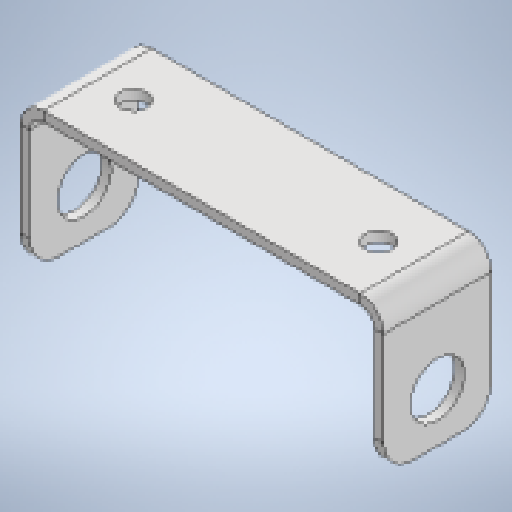
# Autodesk Inventor part: TKS 3525 FDS diam support
Saved by Autodesk Inventor 2025 (Build 290162010, 162A)
## iProperties
Created: 2025-06-24
Part Number: TKS 3525 FDS diam support
Material: Stainless Steel
Document SubType Name: Sheet Metal
Designer: admin
Mass: 14.3451 g
Surface Area: 20.2627 cm^2
Volume: 1.79313 cm^3
Density: 8 g/cm^3
Flat Pattern Width: 12.6404 cm
Flat Pattern Length: 2.2 cm
Flat Pattern Area: 27.8089 cm^2
Sheet Metal Rule: AISI304 2mm Die16
Sheet Metal Width: 126,404 mm
Sheet Metal Length: 22,000 mm
Sheet Metal Area: 2780,888 mm^2
Appearance: Default
Author: user
Autodesk Inventor part; units mm, degrees
ref_plane "YZ Plane" through (0, 0, 0) normal (1, 0, 0) x (0, 1, 0)
ref_plane "XZ Plane" through (0, 0, 0) normal (0, 1, 0) x (-1, 0, 0)
ref_plane "XY Plane" through (0, 0, 0) normal (0, 0, 1) x (1, 0, 0)
sketch "Sketch1" plane through (0, 0, 0) normal (0, 0, 1) x (1, 0, 0)
  line L0 (-35, -11) -> (35, -11)
  line L1 (35, -11) -> (35, 11)
  line L2 (35, 11) -> (-35, 11)
  line L3 (-35, 11) -> (-35, -11)
  line L4 (-35, -11) -> (35, 11) construction
  line L5 (35, -11) -> (-35, 11) construction
  circle A0 centre (-25, 0) radius 2.75
  circle A1 centre (25, 0) radius 2.75
  line L6 (0, 11) -> (0, -18.7198) construction
  point P0 (0, 0)
  dimension "d154" = 70
  dimension "d155" = 22
  dimension "d197" = 50
  dimension "d198" = 5.5
  measures "d154" distance of L1.end L2.end
  measures "d155" distance of L0.end L1.end
  measures "d197" distance of A1.centre A0.centre
  measures "d198" diameter of A0
extrude "Plate5" add sketch "Sketch1" along normal blind 2
sketch "Sketch10" plane through (-37, 11, 2) normal (1, 0, 0) x (0, 1, 0)
  line L0 (-22, 0) -> (0, 0)
  line L1 (0, 0) -> (0, -30)
  line L2 (0, -30) -> (-22, -30)
  line L3 (-22, -30) -> (-22, 0)
  constraints: 8 end point
edge flange "Flange4" height 30 angle 90 thickness 2 bend radius 2.75 thickness toward (1, 0, 0) relief round relief width 2 relief depth 1 corner gap 2.75 corner form 0 edges at (-35, 0, 0) (35, 0, 0) wall of the first edge with corners at (-37, -11, 2) (-37, 11, 2) (-37, 11, -28) (-37, -11, -28)
bend "Bend4"
corner "Corner4"
sketch "Sketch11" plane through (-35, -11, -28) normal (1, 0, 0) x (0, 0, -1)
  line L0 (-25.25, 22) -> (-25.25, 0) construction
  line L1 (-25.25, 0) -> (0, 0) construction
  line L2 (0, 0) -> (0, 22) construction
  line L3 (-25.25, 22) -> (0, 22) construction
  circle A0 centre (-10, 11) radius 5.5
  point P0 (-28, 11)
  point P1 (0, 11)
  dimension "d192" = 11
  dimension "d193" = 10
  constraints: 1 centre point, 1 horizontal alignment, 1 midpoint
  measures "d192" diameter of A0
  measures "d193" distance from line of A0.centre L2
extrude "Cut3" cut sketch "Sketch11" against normal blind 2
mirror "Mirror1" about plane through (0, 0, 0) normal (1, 0, 0) of "Cut3"
fillet "Corner Round3" radius 6 4 edges at (-36, 11, -28) (-36, -11, -28) (36, -11, -28) (36, 11, -28)
body "Solid3"
